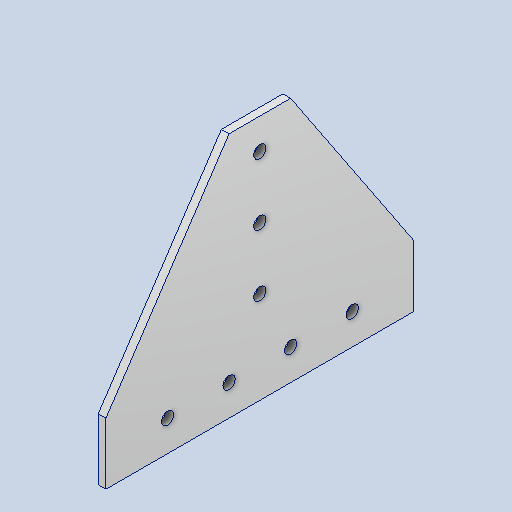
# Autodesk Inventor part: T-Gusset
Saved by Autodesk Inventor 2024 (Build 280153000, 153)
## iProperties
Created: 2023-04-21
Part Number: T-Gusset
Material: Aluminum 6061
Document SubType Name: Modeling
Designer: legom
Density: 2.7 g/cm^3
Appearance: Aluminum - Flat
Author: legom
Autodesk Inventor part; units mm, degrees
ref_plane "YZ Plane" through (0, 0, 0) normal (1, 0, 0) x (0, 1, 0)
ref_plane "XZ Plane" through (0, 0, 0) normal (0, 1, 0) x (-1, 0, 0)
ref_plane "XY Plane" through (0, 0, 0) normal (0, 0, 1) x (1, 0, 0)
sketch "Sketch1" plane through (0, 0, 0) normal (1, 0, 0) x (0, 1, 0)
  line L0 (0, 0) -> (25.4, 0)
  line L1 (25.4, 0) -> (25.4, -127)
  line L2 (25.4, -127) -> (0, -127)
  line L3 (0, -127) -> (0, 0)
  line L4 (101.6, -50.8) -> (25.4, -50.8)
  line L5 (25.4, -50.8) -> (25.4, -76.2)
  line L6 (25.4, -76.2) -> (101.6, -76.2)
  line L7 (101.6, -76.2) -> (101.6, -50.8)
  circle A0 centre (12.7, -25.4) radius 2.5527
  circle A1 centre (12.7, -50.8) radius 2.5527
  circle A2 centre (12.7, -76.2) radius 2.5527
  circle A3 centre (12.7, -101.6) radius 2.5527
  circle A4 centre (88.9, -63.5) radius 2.5527
  circle A5 centre (63.5, -63.5) radius 2.5527
  circle A6 centre (38.1, -63.5) radius 2.5527
  line L8 (25.4, 0) -> (101.6, -50.8)
  line L9 (101.6, -76.2) -> (25.4, -127)
  point P0 (25.4, -63.5)
  dimension "d0" = 25.4
  dimension "d1" = 127
  dimension "d2" = 76.2
  dimension "d3" = 25.4
  dimension "d4" = 5.1054
  dimension "d5" = 25.4
  dimension "d6" = 12.7
  dimension "d9" = 25.4
  dimension "d14" = 5.1054
  dimension "d15" = 12.7
  dimension "d16" = 12.7
  dimension "d19" = 25.4
  constraints: 20 end point, 7 centre point, 4 parallel, 3 horizontal, 2 midpoint, 2 perpendicular, 1 vertical, 10 other
  measures "d0" distance of L1.end L2.end
  measures "d1" distance of L0.end L1.end
  measures "d2" distance of L6.end L5.end
  measures "d3" distance of L5.end L4.end
  measures "d4" diameter of A0
  measures "d5" distance from line of L0 A0.centre
  measures "d6" distance from line of L3 A0.centre
  measures "d9" distance of A0.centre A1.centre
  measures "d14" diameter of A4
  measures "d15" distance from line of L7 A4.centre
  measures "d16" distance from line of L6 A4.centre
  measures "d19" distance of A4.centre A5.centre
extrude "Extrusion1" add sketch "Sketch1" along normal blind 3.175
body "Solid1"
